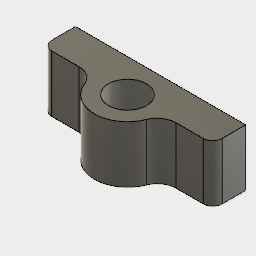
Bearing (Autodesk Fusion 360 design; units mm, degrees)
Autodesk Fusion 360 part; units mm, degrees
sketch "Sketch1" plane through (0, 0, 0) normal (0, 1, 0) x (1, 0, 0)
  line L0 (4.7621, -27) -> (-1, -27)
  line L1 (-3, -25) -> (-3, -20)
  line L2 (-3, -20) -> (33, -20)
  line L3 (33, -20) -> (33, -25)
  line L4 (31, -27) -> (25.2379, -27)
  circle A0 centre (15, -26.9925) radius 4.015
  arc A1 (8.4762, -29.5377) -> (21.5238, -29.5377) centre (15, -26.9925) ccw
  arc A2 (25.2379, -27) -> (21.5238, -29.5377) centre (25.2379, -30.9867) ccw
  line L5 (15, -31.0075) -> (15, -32)
  arc A3 (8.4762, -29.5377) -> (4.7621, -27) centre (4.7621, -30.9867) ccw
  arc A4 (-3, -25) -> (-1, -27) centre (-1, -25) ccw
  arc A5 (31, -27) -> (33, -25) centre (31, -25) ccw
  dimension "d1" = 8.03
  dimension "d2" = 2
  dimension "d3" = 2
  measures "d1" diameter of A0
  measures "d2" radius of A4
  measures "d3" radius of A5
extrude "Extrude1" add sketch "Sketch1" along normal blind 12
named bodies: "Bearing"
